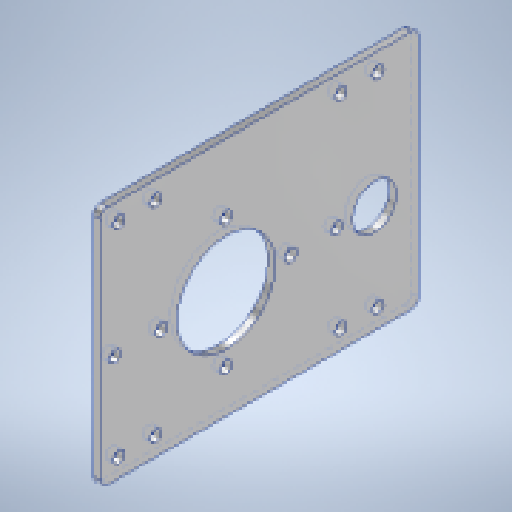
# Autodesk Inventor part: motor
Saved by Autodesk Inventor 2025 (Build 290162000, 162)
## iProperties
Created: 2025-02-25
Part Number: motor
Material: アルミニウム 6061
Document SubType Name: Modeling
Designer: Zhopa
Density: 2.7 g/cm^3
Appearance: アルミニウム - フラット
Mass: 25.9704 g
Surface Area: 107.392 cm^2
Volume: 9.61866 cm^3
Author: Zhopa
Autodesk Inventor part; units mm, degrees
ref_plane "YZ Plane" through (0, 0, 0) normal (1, 0, 0) x (0, 1, 0)
ref_plane "XZ Plane" through (0, 0, 0) normal (0, 1, 0) x (-1, 0, 0)
ref_plane "XY Plane" through (0, 0, 0) normal (0, 0, 1) x (1, 0, 0)
sketch "Sketch1" plane through (0, 0, 0) normal (1, 0, 0) x (0, 1, 0)
  circle A0 centre (0, 0) radius 13.25
  line L0 (36, -46) -> (36, 34)
  line L1 (36, 34) -> (-29, 34)
  line L2 (-29, 34) -> (-29, -46)
  line L3 (-29, -46) -> (36, -46)
  point P0 (0, -17.5)
  point P1 (17.5, 0)
  point P2 (0, 17.5)
  point P3 (-17.5, 0)
  point P4 (0, -30)
  point P5 (0, 30)
  point P6 (31, -41)
  point P7 (31, 29)
  point P8 (-24, 29)
  point P9 (-24, -41)
  dimension "d0" = 26.5
  dimension "d1" = 17.5
  dimension "d4" = 360
  dimension "d6" = 30
  dimension "d9" = 360
  dimension "d15" = 5
  dimension "d16" = 5
  dimension "d17" = 80
  dimension "d18" = 65
  dimension "d28" = 5
  dimension "d29" = 55
  dimension "d30" = 55
  constraints: 8 end point, 3 perpendicular, 1 centre point, 1 coincident, 1 vertical, 8 other
  measures "d0" diameter of A0
  measures "d1" distance of point (0, -17.5) point (0, 0)
  measures "d6" distance of point (0, -30) point (0, 0)
  measures "d15" horizontal distance of L0.start point (31, -41)
  measures "d16" horizontal distance of L0.start point (31, -41)
  measures "d17" distance of L0.start L0.end
  measures "d18" distance of L0.end L1.end
  measures "d28" distance from line of point (31, 29) L1
  measures "d29" distance of point (-24, 29) point (31, 29)
  measures "d30" distance of point (31, -41) point (-24, -41)
extrude "Extrusion1" add sketch "Sketch1" along normal blind 2
hole "Hole1" at (0, 0, -17.5) at (0, 17.5, 0) at (0, 0, 17.5) at (0, -17.5, 0) at (0, 0, -30) at (0, 0, 30) at (0, 31, -41) at (0, 31, 29) at (0, -24, 29) at (0, -24, -41) direction (1, 0, 0) diameter 3.2 depth 43.75 tip angle 118
sketch "Sketch2" plane through (0, 0, 0) normal (-1, 0, 0) x (0, 0, 1)
  circle A0 centre (-40, 0) radius 6
  line L0 (-46, 36) -> (34, 36) projected
  line L1 (-46, 36) -> (-52, 36)
  line L2 (-52, 36) -> (-52, -29)
  line L3 (-52, -29) -> (-46, -29)
  line L4 (-46, -29) -> (-46, 36)
  point P0 (0, 0)
  point P1 (0, 25.1294)
  point P2 (0, -32.6005)
  dimension "d31" = 40
  dimension "d32" = 12
  dimension "d33" = 6
  constraints: 8 end point, 2 parallel, 1 centre point, 1 coincident, 1 horizontal, 1 perpendicular
  measures "d31" distance of point (-40, 0) point (0, 0)
  measures "d32" diameter of A0
  measures "d33" distance of L3.end L2.end
extrude "Extrusion2" add sketch "Sketch2" against normal blind 2 contours L4 L3 L2 L1
extrude "Extrusion3" cut sketch "Sketch2" against normal blind 2 contours A0
sketch "Sketch3" plane through (2, 0, 0) normal (1, 0, 0) x (0, 0, -1)
  circle A0 centre (41, 31) radius 1.6 projected
  circle A1 centre (-29, 31) radius 1.6 projected
  circle A2 centre (-29, -24) radius 1.6 projected
  circle A3 centre (41, -24) radius 1.6 projected
  point P0 (0, 0)
  point P1 (-19, 31)
  point P2 (31, 31)
  point P3 (-19, -24)
  point P4 (31, -24)
  dimension "d38" = 10
  dimension "d39" = 10
  dimension "d40" = 10
  dimension "d41" = 10
  measures "d38" distance of point (31, 31) A0.centre
  measures "d39" distance of A1.centre point (-19, 31)
  measures "d40" distance of A2.centre point (-19, -24)
  measures "d41" distance of A3.centre point (31, -24)
hole "Hole2" at (2, 31, 19) at (2, 31, -31) at (2, -24, 19) at (2, -24, -31) direction (-1, 0, 0) diameter 3.2 depth 43.75 tip angle 118
fillet "Fillet1" radius 2 4 edges at (1, 36, 34) (1, 36, -52) (1, -29, -52) (1, -29, 34)
body "Solid1"
